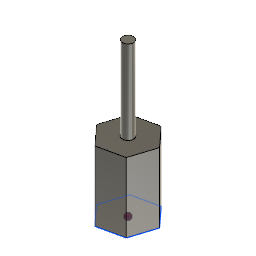
Polygon Wedge Print (Autodesk Fusion 360 design; units mm, degrees)
Autodesk Fusion 360 part; units mm, degrees
sketch "Sketch1" plane through (0, 0, 0) normal (0, 0, 1) x (1, 0, 0)
  line L0 (2.5647, -2.804) -> (3.7107, 0.819)
  line L1 (3.7107, 0.819) -> (1.146, 3.6231)
  line L2 (1.146, 3.6231) -> (-2.5647, 2.804)
  line L3 (-2.5647, 2.804) -> (-3.7107, -0.819)
  line L4 (-3.7107, -0.819) -> (-1.146, -3.6231)
  line L5 (-1.146, -3.6231) -> (2.5647, -2.804)
  dimension "d1" = 3.8
  measures "d1" distance of L0.start origin
extrude "Extrude1" add sketch "Sketch1" along normal blind 10
sketch "Sketch2" plane through (0, 0, 10) normal (0, 0, 1) x (-1, 0, 0)
  line L0 (1.146, 3.6231) -> (-2.5647, 2.804)
  line L1 (-2.5647, 2.804) -> (-3.7107, -0.819)
  line L2 (-3.7107, -0.819) -> (-1.146, -3.6231)
  line L3 (-1.146, -3.6231) -> (2.5647, -2.804)
  line L4 (2.5647, -2.804) -> (3.7107, 0.819)
  line L5 (3.7107, 0.819) -> (1.146, 3.6231)
  circle A0 centre (0, 0) radius 0.8
  dimension "d6" = 1.6
  constraint coincident A0.centre origin
  measures "d6" diameter of A0
extrude "Extrude2" add sketch "Sketch2" along normal blind 12 contours A0
equation "d1 = polygon_side"
equation "d2 = polygon_height"
equation "polygon_side = 3.8 mm"
equation "polygon_height = 10 mm"
equation "d6 = cylinder_radius * 2"
equation "cylinder_radius = 0.8 mm"
equation "cylinder_height = 12 mm"
equation "d9 = cylinder_height"
